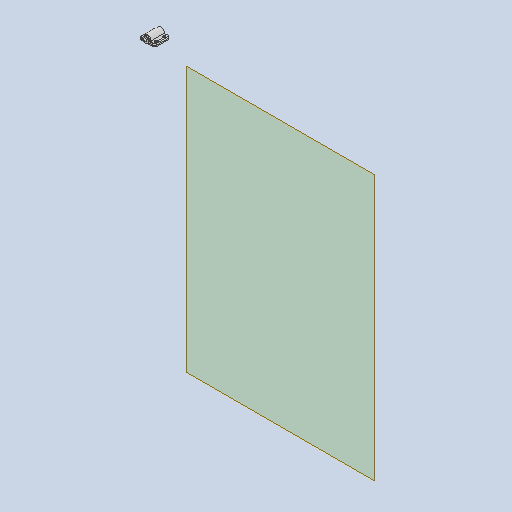
# Autodesk Inventor part: RollerHolder
Saved by Autodesk Inventor 2023 (Build 270158000, 158)
## iProperties
Created: 2023-08-15
Part Number: RollerHolder
Material: Generic
Document SubType Name: Modeling
Designer: Felix
Density: 1 g/cm^3
Appearance: Default
Author: Felix
Autodesk Inventor part; units mm, degrees
ref_plane "YZ Plane" through (0, 0, 0) normal (1, 0, 0) x (0, 1, 0)
ref_plane "XZ Plane" through (0, 0, 0) normal (0, 1, 0) x (-1, 0, 0)
ref_plane "Work Plane1" through (55.3183, -93.0267, 219.4595) normal (0, 0, -1) x (-1, 0, 0)
sketch "Sketch1" plane through (55.3183, -93.0267, 219.4595) normal (0, 0, -1) x (-1, 0, 0)
  line L0 (-310, 367) -> (310, 367) construction
  circle A0 centre (289.3, 376) radius 4 construction
  arc A1 (289.3, 367) -> (297.3623, 372) centre (289.3, 376) ccw construction
  line L1 (270.3, 367) -> (308.3, 367)
  line L2 (308.3, 367) -> (308.3, 370)
  line L3 (306.3, 372) -> (302.3, 372)
  line L4 (270.3, 370) -> (270.3, 367)
  arc A2 (281.2377, 372) -> (289.3, 367) centre (289.3, 376) ccw construction
  arc A3 (298.3, 376) -> (280.3, 376) centre (289.3, 376) ccw
  line L5 (297.3623, 372) -> (281.2377, 372) construction
  line L6 (276.3, 372) -> (272.3, 372)
  arc A4 (276.3, 372) -> (280.3, 376) centre (276.3, 376) ccw
  arc A5 (298.3, 376) -> (302.3, 372) centre (302.3, 376) ccw
  arc A6 (272.3, 372) -> (270.3, 370) centre (272.3, 370) ccw
  arc A7 (308.3, 370) -> (306.3, 372) centre (306.3, 370) ccw
  point P0 (55.3183, 93.0267)
  point P1 (270.3, 372)
  dimension "d10" = 10
  dimension "d11" = 10
  dimension "d12" = 5
  dimension "d14" = 2
  constraints: 16 point on circle, 12 end point, 10 tangent, 7 centre point, 6 point on line, 4 parallel, 2 equal radius, 1 coincident, 1 horizontal, 1 horizontal alignment, 1 midpoint, 1 perpendicular
  measures "d10" distance edge to line of A1 L4
  measures "d11" distance edge to line of A1 L2
  measures "d12" distance of point (270.3, 372) L1.start
  measures "d14" radius of A6
ref_plane "Work Plane2" through (-254.6817, 268.1733, 259.4595) normal (0, 0, 1) x (1, 0, 0)
extrude "Extrusion1" add sketch "Sketch1" against normal up to surface (40 mm away)
sketch "Sketch2" plane through (-220.9817, 278.9733, 219.4595) normal (0, 1, 0) x (1, 0, 0)
  line L0 (-33.7, -29.9) -> (-33.7, -30.1) construction
  line L1 (-33.7, -9.9) -> (-33.7, -10.1) construction
  line L2 (-33.7, -30) -> (52.868, -30) construction
  line L3 (-33.7, -10) -> (52.3947, -10) construction
  line L4 (6, -40) -> (-32, -40) construction
  line L5 (-32, 0) -> (-32, -40) construction
  line L6 (6, 0) -> (-32, 0) construction
  line L7 (6, 0) -> (6, -40) construction
  line L8 (1, -40) -> (1, 0) construction
  line L9 (-27, -40) -> (-27, 0) construction
  line L10 (-26, 0) -> (-22, 0) construction
  point P0 (220.9817, 219.4595)
  point P1 (1, -30)
  point P2 (-27, -30)
  point P3 (-27, -10)
  point P4 (1, -10)
  dimension "d17" = 5
  dimension "d18" = 5
  constraints: 12 point on line, 8 end point, 2 horizontal, 2 midpoint, 2 perpendicular
  measures "d17" distance between parallel lines of L7 L8
  measures "d18" distance between parallel lines of L5 L9
hole "Hole1" at (-219.9817, 278.9733, 249.4595) at (-219.9817, 278.9733, 229.4595) at (-247.9817, 278.9733, 229.4595) at (-247.9817, 278.9733, 249.4595) direction (0, -1, 0) diameter 5 end through all
sketch "Sketch3" plane through (-250.9817, 278.9733, 259.4595) normal (0, 1, 0) x (1, 0, 0)
  circle A0 centre (3, 10) radius 4 projected
  circle A1 centre (3, 10) radius 2.5 projected
  circle A2 centre (31, 10) radius 4 projected
  circle A3 centre (31, 10) radius 2.5 projected
  circle A4 centre (31, 30) radius 4 projected
  circle A5 centre (31, 30) radius 2.5 projected
  circle A6 centre (3, 30) radius 4 projected
  circle A7 centre (3, 30) radius 2.5 projected
  point P0 (250.9817, 259.4595)
extrude "Extrusion2" cut sketch "Sketch3" along normal through all contours A0 | A1 | A2 | A3 | A4 | A5 | A6 | A7
sketch "Sketch4" plane through (55.3183, -93.0267, 219.4595) normal (0, 0, -1) x (-1, 0, 0)
  arc A0 (298.3, 376) -> (280.3, 376) centre (289.3, 376) ccw projected
  point P0 (55.3183, 93.0267)
  constraints: 1 coincident
hole "Hole2" at (-233.9817, 282.9733, 219.4595) direction (0, 0, 1) diameter 8.4 end through all counterbore diameter 18.01 counterbore depth 5.68 clearance for "Hex Head Bolt" size "M8" standard "Ansi Metric M Profile"
sketch "Sketch5" plane through (55.3183, -93.0267, 219.4595) normal (0, 0, -1) x (-1, 0, 0)
  arc A0 (280.2965, 375.8336) -> (289, 367) centre (289.3, 376) ccw projected
  arc A1 (276.3, 372) -> (280.2965, 375.8336) centre (276.3, 376) ccw projected
  line L0 (276.3, 372) -> (272.3, 372) projected
  arc A2 (272.3, 372) -> (270.3, 370) centre (272.3, 370) ccw projected
  line L1 (270.3, 370) -> (270.3, 367) projected
  line L2 (270.3, 367) -> (289, 367) projected
  arc A3 (289.6, 367) -> (298.3035, 375.8336) centre (289.3, 376) ccw projected
  line L3 (289.6, 367) -> (308.3, 367) projected
  line L4 (308.3, 367) -> (308.3, 370) projected
  arc A4 (308.3, 370) -> (306.3, 372) centre (306.3, 370) ccw projected
  line L5 (306.3, 372) -> (302.3, 372) projected
  arc A5 (298.3035, 375.8336) -> (302.3, 372) centre (302.3, 376) ccw projected
  point P0 (55.3183, 93.0267)
extrude "Extrusion3" cut sketch "Sketch5" against normal blind 2
sketch "Sketch6" plane through (55.3183, -93.0267, 221.4595) normal (0, 0, -1) x (-1, 0, 0)
  arc A0 (272.3, 372) -> (270.3, 370) centre (272.3, 370) ccw projected
  line L0 (270.3, 367) -> (270.3, 370) projected
  line L1 (289, 367) -> (270.3, 367) projected
  arc A1 (280.2965, 375.8336) -> (289, 367) centre (289.3, 376) ccw projected
  arc A2 (276.3, 372) -> (280.2965, 375.8336) centre (276.3, 376) ccw construction
  line L2 (272.3, 372) -> (276.3, 372) construction
  arc A3 (308.3, 370) -> (306.3, 372) centre (306.3, 370) ccw projected
  line L3 (302.3, 372) -> (306.3, 372) construction
  arc A4 (298.3035, 375.8336) -> (302.3, 372) centre (302.3, 376) ccw projected
  arc A5 (289.6, 367) -> (298.3035, 375.8336) centre (289.3, 376) ccw projected
  line L4 (308.3, 367) -> (289.6, 367) projected
  line L5 (308.3, 370) -> (308.3, 367) projected
  line L6 (280.3, 370) -> (280.3, 367)
  line L7 (270.3, 367) -> (308.3, 367) projected
  arc A6 (276.3, 372) -> (280.3, 376) centre (276.3, 376) ccw projected
  line L8 (272.3, 372) -> (276.3, 372) projected
  line L9 (278.3, 372) -> (272.3, 372)
  arc A7 (280.3, 370) -> (278.3, 372) centre (278.3, 370) ccw
  line L10 (289.3, 376) -> (289.3, 367) construction
  line L11 (289.6, 367) -> (289, 367) construction
  line L12 (298.3, 370) -> (298.3, 367)
  line L13 (300.3, 372) -> (306.3, 372)
  arc A8 (300.3, 372) -> (298.3, 370) centre (300.3, 370) ccw
  point P0 (55.3183, 93.0267)
  point P1 (280.3, 372)
  point P2 (298.3, 372)
  point P3 (276.3, 372)
  dimension "d38" = 2
  constraints: 10 end point, 7 point on line, 5 point on circle, 5 symmetric about line, 2 centre point, 2 tangent, 1 horizontal, 1 midpoint, 1 perpendicular, 1 other
  measures "d38" radius of A7
extrude "Extrusion4" cut sketch "Sketch6" against normal up to surface (3.68 mm away) contours A6 A1 L1 L6 A7 L9 | L13 A8 L12 L4 A5 A4
sketch "Sketch7" plane through (-252.9817, 273.9733, 259.4595) normal (0, -1, 0) x (1, 0, 0)
  line L0 (10, -34.32) -> (28, -34.32) construction
  line L1 (28, -34.32) -> (28, -38) projected
  line L2 (28, -38) -> (38, -38) projected
  line L3 (38, -38) -> (38, 0) construction
  line L4 (38, 0) -> (0, 0) projected
  line L5 (0, -38) -> (0, 0) projected
  line L6 (0, -38) -> (10, -38) projected
  line L7 (10, -38) -> (10, -34.32) projected
  circle A0 centre (5, -10) radius 2.5 construction
  circle A1 centre (33, -30) radius 2.5 construction
  circle A2 centre (33, -10) radius 2.5 construction
  circle A3 centre (5, -30) radius 2.5 construction
  line L8 (38, -38) -> (38, 0) projected
  line L9 (10, 0) -> (28, 0) projected
  line L10 (33, -38) -> (33, -38)
  line L11 (28, -33) -> (28, -5)
  line L12 (33, 0) -> (33, 0)
  line L13 (38, -5) -> (38, -33)
  line L14 (5, -38) -> (5, -38)
  line L15 (0, -33) -> (0, -5)
  line L16 (5, 0) -> (5, 0)
  line L17 (10, -5) -> (10, -33)
  arc A4 (33, -38) -> (38, -33) centre (33, -33) ccw
  arc A5 (28, -33) -> (33, -38) centre (33, -33) ccw
  arc A6 (5, -38) -> (10, -33) centre (5, -33) ccw
  arc A7 (0, -33) -> (5, -38) centre (5, -33) ccw
  arc A8 (5, 0) -> (0, -5) centre (5, -5) ccw
  arc A9 (10, -5) -> (5, 0) centre (5, -5) ccw
  line L18 (28, -34.32) -> (28, -33)
  line L19 (28, -34.32) -> (28, 0) projected
  line L20 (30, -34.32) -> (28, -34.32) construction
  line L21 (28, -34.32) -> (28.1774, -34.32)
  line L22 (28, -34.32) -> (10, -34.32) projected
  line L23 (10, -34.32) -> (9.8226, -34.32)
  arc A10 (38, -5) -> (33, 0) centre (33, -5) ccw
  arc A11 (33, 0) -> (28, -5) centre (33, -5) ccw
  point P0 (252.9817, -259.4595)
  point P1 (0, -5)
  point P2 (33, 0)
  point P3 (38, -5)
  point P4 (33, -38)
  point P5 (33, -38)
  point P6 (33, -38)
  point P7 (38, -33)
  dimension "d41" = 5
  dimension "d42" = 5
  constraints: 22 end point, 18 point on circle, 16 tangent, 10 point on line, 8 centre point, 6 equal radius, 4 parallel, 2 horizontal, 2 perpendicular, 1 collinear
  measures "d41" radius of A4
  measures "d42" radius of A10
extrude "Extrusion5" cut sketch "Sketch7" against normal through all contours L21 A5 L2 L1 | L7 L6 A6 L23 | A4 L8 L2 | L4 L8 A10 | L6 L5 A7 | A8 L5 L4
sketch "Sketch8" plane through (-233.9817, 282.9733, 259.4595) normal (0, 0, 1) x (1, 0, 0)
  line L0 (-14, -4) -> (-14, -9) construction
  line L1 (14, -9) -> (-14, -9) construction
  line L2 (14, -4) -> (14, -9) construction
  line L3 (13, -4) -> (14, -4) construction
  arc A0 (9, 0) -> (13, -4) centre (13, 0) ccw construction
  arc A1 (9, 0) -> (-9, 0) centre (0, 0) ccw construction
  arc A2 (-13, -4) -> (-9, 0) centre (-13, 0) ccw construction
  line L4 (-14, -4) -> (-13, -4) construction
  circle A3 centre (0, 0) radius 4.2 projected
  circle A4 centre (0, 0) radius 7.5
  point P0 (233.9817, -282.9733)
  dimension "d45" = 15
  constraints: 1 centre point, 1 coincident
  measures "d45" diameter of A4
extrude "Extrusion6" add sketch "Sketch8" along normal blind 4
fillet "Fillet1" radius 2 1 edges at (-241.4817, 282.9733, 259.4595)
fillet "Fillet2" radius 2 9 edges at (-223.1501, 279.612, 259.4595) (-220.4817, 278.9733, 259.4595) (-218.4006, 278.9733, 259.2029) (-215.4262, 278.2304, 256.5204) (-244.8133, 279.612, 259.4595) (-247.4817, 278.9733, 259.4595) (-249.5628, 278.9733, 259.2029) (-252.5373, 278.2304, 256.5202) (-233.9817, 291.9733, 259.4595)
equation "\"d11\" = d10"
body "Solid1"
